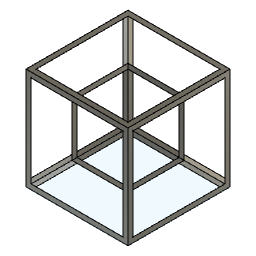
Tesseract (Autodesk Fusion 360 design; units mm, degrees)
Autodesk Fusion 360 part; units mm, degrees
sketch "Sketch1" plane through (0, 0, 0) normal (0, 0, 1) x (1, 0, 0)
  line L0 (63.5, 63.5) -> (-63.5, 63.5)
  line L1 (-63.5, 63.5) -> (-63.5, -63.5)
  line L2 (-63.5, -63.5) -> (63.5, -63.5)
  line L3 (63.5, -63.5) -> (63.5, 63.5)
  line L4 (63.5, 63.5) -> (-63.5, -63.5) construction
  line L5 (-63.5, 63.5) -> (63.5, -63.5) construction
  constraint horizontal L0
  constraint perpendicular L0 L1
  constraint parallel L0 L2
  constraint parallel L1 L3
  constraint coincident L4 origin
  constraint coincident L5 origin
extrude "Extrude1" add sketch "Sketch1" along normal blind 127
sketch "Sketch2" plane through (0, 0, 127) normal (0, 0, 1) x (-1, 0, 0)
  line L0 (-63.5, 63.5) -> (-63.5, -63.5)
  line L1 (-63.5, -63.5) -> (63.5, -63.5)
  line L2 (63.5, -63.5) -> (63.5, 63.5)
  line L3 (63.5, 63.5) -> (-63.5, 63.5)
  line L4 (31.75, 31.75) -> (-31.75, 31.75)
  line L5 (-31.75, 31.75) -> (-31.75, -31.75)
  line L6 (-31.75, -31.75) -> (31.75, -31.75)
  line L7 (31.75, -31.75) -> (31.75, 31.75)
  dimension "d3" = -31.75
sketch "Sketch3" plane through (0, -63.5, 0) normal (0, -1, 0) x (1, 0, 0)
  line L0 (-63.5, 0) -> (63.5, 0)
  line L1 (63.5, 0) -> (63.5, 127)
  line L2 (63.5, 127) -> (-63.5, 127)
  line L3 (-63.5, 127) -> (-63.5, 0)
  line L4 (-31.75, 31.75) -> (31.75, 31.75)
  line L5 (31.75, 31.75) -> (31.75, 95.25)
  line L6 (31.75, 95.25) -> (-31.75, 95.25)
  line L7 (-31.75, 95.25) -> (-31.75, 31.75)
  dimension "d4" = -31.75
sketch "Sketch4" plane through (0, 0, 0) normal (0, 0, -1) x (1, 0, 0)
  line L0 (63.5, -63.5) -> (63.5, 63.5)
  line L1 (63.5, 63.5) -> (-63.5, 63.5)
  line L2 (-63.5, 63.5) -> (-63.5, -63.5)
  line L3 (-63.5, -63.5) -> (63.5, -63.5)
sketch "Sketch5" plane through (-63.5, 0, 0) normal (-1, 0, 0) x (0, -1, 0)
  line L0 (-63.5, 0) -> (63.5, 0)
  line L1 (63.5, 0) -> (63.5, 127)
  line L2 (63.5, 127) -> (-63.5, 127)
  line L3 (-63.5, 127) -> (-63.5, 0)
  line L4 (-31.75, 31.75) -> (31.75, 31.75)
  line L5 (31.75, 31.75) -> (31.75, 95.25)
  line L6 (31.75, 95.25) -> (-31.75, 95.25)
  line L7 (-31.75, 95.25) -> (-31.75, 31.75)
  dimension "d5" = -31.75
extrude "Extrude2" cut sketch "Sketch2" against normal blind 127 contours L4 L5 L6 L7
extrude "Extrude3" cut sketch "Sketch5" against normal blind 127 contours L4 L5 L6 L7
extrude "Extrude4" cut sketch "Sketch3" against normal blind 127 contours L4 L5 L6 L7
chamfer "Chamfer1" distance 25.4 angle 45 4 edges at (0, -63.5, 95.25) (31.75, -63.5, 63.5) (0, -63.5, 31.75) (-31.75, -63.5, 63.5)
chamfer "Chamfer2" distance 25.4 angle 45 4 edges at (-63.5, 31.75, 63.5) (-63.5, 0, 95.25) (-63.5, -31.75, 63.5) (-63.5, 0, 31.75)
chamfer "Chamfer3" distance 25.4 angle 45 4 edges at (31.75, 63.5, 63.5) (0, 63.5, 95.25) (-31.75, 63.5, 63.5) (0, 63.5, 31.75)
chamfer "Chamfer4" distance 25.4 angle 45 4 edges at (63.5, 0, 95.25) (63.5, 31.75, 63.5) (63.5, 0, 31.75) (63.5, -31.75, 63.5)
chamfer "Chamfer5" distance 25.4 angle 45 4 edges at (-31.75, 0, 127) (0, 31.75, 127) (31.75, 0, 127) (0, -31.75, 127)
chamfer "Chamfer6" distance 25.4 angle 45 4 edges at (31.75, 0, 0) (0, 31.75, 0) (-31.75, 0, 0) (0, -31.75, 0)
extrude "Extrude5" cut 1 faces at (-55.0333, 10.5833, 112.1833) along direction (0.707107, 0, 0.707107) blind 12.7
extrude "Extrude6" cut 1 faces at (-55.0333, 10.5833, 14.8167) along direction (0.707107, 0, -0.707107) blind 12.7
extrude "Extrude7" cut 1 faces at (-10.5833, -55.0333, 14.8167) along direction (0, 0.707107, -0.707107) blind 12.7
extrude "Extrude8" cut 1 faces at (-10.5833, -55.0333, 112.1833) along direction (0, 0.707107, 0.707107) blind 12.7
extrude "Extrude9" cut 1 faces at (55.0333, 10.5833, 14.8167) along direction (-0.707107, 0, -0.707107) blind 12.7
extrude "Extrude10" cut 1 faces at (55.0333, -10.5833, 112.1833) along direction (-0.707107, 0, 0.707107) blind 12.7
extrude "Extrude11" cut 1 faces at (-10.5833, 55.0333, 14.8167) along direction (0, -0.707107, -0.707107) blind 12.7
extrude "Extrude12" cut 1 faces at (10.5833, 55.0333, 112.1833) along direction (0, -0.707107, 0.707107) blind 12.7
extrude "Extrude13" cut 1 faces at (48.6833, 55.0333, 74.0833) along direction (0.707107, -0.707107, 0) blind 12.7
extrude "Extrude14" cut 1 faces at (-48.6833, 55.0333, 74.0833) along direction (-0.707107, -0.707107, 0) blind 12.7
extrude "Extrude15" cut 1 faces at (-48.6833, -55.0333, 52.9167) along direction (-0.707107, 0.707107, 0) blind 12.7
extrude "Extrude16" cut 1 faces at (48.6833, -55.0333, 74.0833) along direction (0.707107, 0.707107, 0) blind 12.7
